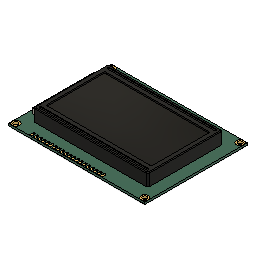
model (Autodesk Fusion 360 design; units mm, degrees)
Autodesk Fusion 360 part; units mm, degrees
note: some values were not read from the file. Set by a fixed rule: which face or edge a step refers to.
sketch "Sketch1" plane through (0, 0, 0) normal (0, 1, 0) x (1, 0, 0)
  line L0 (46.5, 35) -> (-46.5, 35)
  line L1 (-46.5, 35) -> (-46.5, -35)
  line L2 (-46.5, -35) -> (46.5, -35)
  line L3 (46.5, -35) -> (46.5, 35)
  circle A0 centre (-44, 32.5) radius 1.5
  circle A1 centre (44, 32.5) radius 1.5
  circle A2 centre (-44, -32.5) radius 1.5
  circle A3 centre (44, -32.5) radius 1.5
  line L4 (39, 25.5) -> (-39, 25.5)
  line L5 (-39, 25.5) -> (-39, -25.5)
  line L6 (-39, -25.5) -> (39, -25.5)
  line L7 (39, -25.5) -> (39, 25.5)
  line L8 (44, 21.25) -> (39, 21.25)
  line L9 (44, -21.25) -> (39, -21.25)
  line L10 (44, 21.25) -> (44, -21.25)
  dimension "d1" = 93
  dimension "d2" = 70
  dimension "d3" = 88
  dimension "d4" = 65
  dimension "d5" = 3
  dimension "d6" = 3
  dimension "d7" = 3
  dimension "d8" = 3
  dimension "d9" = 78
  dimension "d10" = 51
  constraint horizontal L0
  constraint perpendicular L0 L1
  constraint parallel L0 L2
  constraint parallel L1 L3
  constraint horizontal L4
  constraint perpendicular L4 L5
  constraint parallel L4 L6
  constraint parallel L5 L7
  constraint coincident L7 L8.end
  constraint perpendicular L7 L8
  constraint perpendicular L8 L10
  measures "d1" distance of L1.end L2.end
  measures "d2" distance of L0.end L1.end
  measures "d3" distance of A2.centre A3.centre
  measures "d4" distance of A0.centre A2.centre
  measures "d5" diameter of A0
  measures "d6" diameter of A1
  measures "d7" diameter of A2
  measures "d8" diameter of A3
  measures "d9" distance of L5.end L6.end
  measures "d10" distance of L4.end L5.end
extrude "Extrude1" add sketch "Sketch1" against normal blind 1.5 contours L0 L1 L2 L3 | L4 L5 L6 L7 | L7 L8 L9 L10 makes body 1
extrude "Extrude2" add sketch "Sketch1" along normal blind 8.5 contours L4 L5 L6 L7 bodies 1
extrude "Extrude3" add sketch "Sketch1" along normal blind 3.5 separate body contours L7 L8 L9 L10 makes body 2
extrude "Extrude4" cut 1 faces at (39, 1.1667, 7.0833) along direction (-1, 0, 0) blind 74 on bodies 2 bodies 1
split "Split1" by plane through (0, 0, 0) normal (0, 1, 0) bodies 1 makes body 3 at (-13, 8.5, -8.5)
extrude "Extrude5" cut 1 faces at (14.3333, 3.5, 7.0833) along direction (0, 1, 0) blind 1 on bodies 3 bodies 3
extrude "Extrude6" cut 1 faces at (14.3333, 1.5, -21.25) along direction (0, 0, -1) blind 1 on bodies 3 bodies 3
extrude "Extrude7" cut 1 faces at (14.3333, 1.5, 21.25) along direction (0, 0, 1) blind 1 on bodies 3 bodies 3
extrude "Extrude8" cut 1 faces at (-35, 1.5, -7.4167) along direction (-1, 0, 0) blind 0.75 on bodies 3 bodies 3
extrude "Extrude9" add 1 faces at (39, 1.1667, 7.0833) along direction (-1, 0, 0) blind 73.75 on bodies 2 bodies 2
sketch "Sketch2" plane through (0, 8.5, 0) normal (0, 1, 0) x (-1, 0, 0)
  line L0 (-39, 25.5) -> (-39, -25.5)
  line L1 (-39, -25.5) -> (39, -25.5)
  line L2 (39, -25.5) -> (39, 25.5)
  line L3 (39, 25.5) -> (-39, 25.5)
  line L4 (-35, -20) -> (35, -20)
  line L5 (36, -19) -> (36, 19)
  line L6 (35, 20) -> (-35, 20)
  line L7 (-36, 19) -> (-36, -19)
  line L8 (-36, -20) -> (36, 20) construction
  line L9 (36, -20) -> (-36, 20) construction
  arc A0 (35, -20) -> (36, -19) centre (35, -19) ccw
  arc A1 (36, 19) -> (35, 20) centre (35, 19) ccw
  arc A2 (-35, 20) -> (-36, 19) centre (-35, 19) ccw
  arc A3 (-36, -19) -> (-35, -20) centre (-35, -19) ccw
  dimension "d31" = 72
  dimension "d32" = 40
  dimension "d33" = 1
  constraint horizontal L4
  constraint perpendicular L4 L5
  constraint parallel L4 L6
  constraint parallel L5 L7
  constraint coincident L8 origin
  constraint coincident L9 origin
  constraint coincident L9.start L5
  constraint coincident L9.start L4
  constraint tangent L5 A0
  constraint tangent L4 A0
  constraint coincident L8.end L5
  constraint coincident L8.end L6
  constraint tangent L5 A1
  constraint tangent L6 A1
  constraint equal A0 A1
  constraint coincident L9.end L6
  constraint coincident L9.end L7
  constraint tangent L6 A2
  constraint tangent L7 A2
  constraint equal A0 A2
  constraint coincident L8.start L7
  constraint coincident L8.start L4
  constraint tangent L7 A3
  constraint tangent L4 A3
  constraint equal A0 A3
  measures "d31" distance of L8.end L9.end
  measures "d32" distance of L9.start L8.end
  measures "d33" radius of A0
extrude "Extrude10" cut sketch "Sketch2" against normal blind 1 contours L4 L5 L6 L7 A0 A1 A2 A3 bodies 3
chamfer "Chamfer1" distance 1 angle 45 4 edges at (-39, 4.25, 25.5) (39, 4.25, 25.5) (-39, 4.25, -25.5) (39, 4.25, -25.5) on bodies 3
fillet "Fillet1" radius 0.5 8 edges at (39, 8.5, 0) (0, 8.5, 25.5) (38.5, 8.5, 25) (38.5, 8.5, -25) (0, 8.5, -25.5) (-38.5, 8.5, 25) (-39, 8.5, 0) (-38.5, 8.5, -25) on bodies 3
sketch "Sketch3" plane through (0, 8.5, 0) normal (0, 1, 0) x (-1, 0, 0)
  line L0 (35, -20) -> (-35, -20)
  arc A0 (-36, -19) -> (-35, -20) centre (-35, -19) ccw
  line L1 (-36, -19) -> (-36, 19)
  arc A1 (-35, 20) -> (-36, 19) centre (-35, 19) ccw
  line L2 (-35, 20) -> (35, 20)
  arc A2 (36, 19) -> (35, 20) centre (35, 19) ccw
  line L3 (36, 19) -> (36, -19)
  arc A3 (35, -20) -> (36, -19) centre (35, -19) ccw
  line L4 (38.5, -24.2929) -> (38.5, 24.2929)
  line L5 (38.5, 24.2929) -> (37.7929, 25)
  line L6 (37.7929, 25) -> (-37.7929, 25)
  line L7 (-37.7929, 25) -> (-38.5, 24.2929)
  line L8 (-38.5, 24.2929) -> (-38.5, -24.2929)
  line L9 (-38.5, -24.2929) -> (-37.7929, -25)
  line L10 (-37.7929, -25) -> (37.7929, -25)
  line L11 (37.7929, -25) -> (38.5, -24.2929)
  line L12 (-36.5, -23.95) -> (36.5, -23.95)
  arc A4 (36.5, -23.95) -> (36.5, -22.45) centre (36.5, -23.2) ccw
  line L13 (36.5, -22.45) -> (-36.5, -22.45)
  arc A5 (-36.5, -22.45) -> (-36.5, -23.95) centre (-36.5, -23.2) ccw
  line L14 (-36.5, -23.2) -> (36.5, -23.2) construction
  line L15 (36.5, 23.95) -> (-36.5, 23.95)
  arc A6 (-36.5, 23.95) -> (-36.5, 22.45) centre (-36.5, 23.2) ccw
  line L16 (-36.5, 22.45) -> (36.5, 22.45)
  arc A7 (36.5, 22.45) -> (36.5, 23.95) centre (36.5, 23.2) ccw
  point P0 (0, -23.2)
  dimension "d39" = 1.5
  dimension "d40" = 1.5
  constraint tangent L12 A4
  constraint tangent A4 L13
  constraint parallel L12 L13
  constraint tangent L13 A5
  constraint tangent L12 A5
  constraint perpendicular L4 L14
  constraint midpoint L14 P0
  constraint tangent L15 A6
  constraint tangent A6 L16
  constraint parallel L15 L16
  constraint tangent L16 A7
  constraint tangent L15 A7
  measures "d39" diameter of A4
  measures "d40" diameter of A6
extrude "Extrude11" cut sketch "Sketch3" against normal blind 0.5 contours L12 A4 L13 A5 | L15 A6 L16 A7 bodies 3
cylinder "CylinderPrimitive1" add diameter 5 height 0.25 placed x (1, 0, 0) y (0, 0, -1) z (0, 1, 0) at (44, 0, 32.5) separate body makes body 4
extrude "Extrude12" add 1 faces at (43.4804, 0.25, 32.0179) along direction (0, -1, 0) blind 2 separate body on bodies 4 makes body 5
copy_body "CopyPasteBodies1" bodies 5 makes body 6
move_body "Move1" bodies 6 to x (1, 0, 0) y (0, 1, 0) z (0, 0, 1) at (-88, 0, 0)
copy_body "CopyPasteBodies2" bodies 6 5 makes body 7 makes body 8
move_body "Move2" bodies 7 8 to x (1, 0, 0) y (0, 1, 0) z (0, 0, 1) at (0, 0, -65)
combine "Combine1" operation add target body 8 tool bodies 7 6 5 4 1
cylinder "CylinderPrimitive2" cut diameter 3 height -2 placed x (1, 0, 0) y (0, 0, -1) z (0, 1, 0) at (-44, 0.25, 32.5) bodies 8
cylinder "CylinderPrimitive3" cut diameter 3 height -2 placed x (1, 0, 0) y (0, 0, -1) z (0, 1, 0) at (44, 0.25, 32.5) bodies 8
cylinder "CylinderPrimitive4" cut diameter 3 height -2 placed x (1, 0, 0) y (0, 0, -1) z (0, 1, 0) at (44, 0.25, -32.5) bodies 8
cylinder "CylinderPrimitive5" cut diameter 3 height -2 placed x (1, 0, 0) y (0, 0, -1) z (0, 1, 0) at (-44, 0.25, -32.5) bodies 8
extrude "Extrude13" cut 4 faces at (-41.8482, 0.25, -32.3013) (46.1518, 0.25, -32.3013) (46.1518, 0.25, 32.6987) (-41.8482, 0.25, 32.6987) along direction (0, -1, 0) blind 0.15 on bodies 8 bodies 8
extrude "Extrude14" cut 4 faces at (46.1518, -1.75, -32.3013) (46.1518, -1.75, 32.6987) (-41.8482, -1.75, 32.6987) (-41.8482, -1.75, -32.3013) along direction (0, 1, 0) blind 0.15 on bodies 8 bodies 8
move_body "Move3" bodies 2 8 3 to x (-1, 0, 0) y (0, 1, 0) z (0, 0, -1) at (0, 0, 0)
sketch "Sketch9" plane through (0, 0, 0) normal (0, 1, 0) x (-1, 0, 0)
  arc A0 (46.5, -32.5) -> (44, -35) centre (44, -32.5) ccw
  line L0 (46.5, -32.5) -> (46.5, 32.5)
  arc A1 (44, 35) -> (46.5, 32.5) centre (44, 32.5) ccw
  line L1 (44, 35) -> (-44, 35)
  arc A2 (-46.5, 32.5) -> (-44, 35) centre (-44, 32.5) ccw
  line L2 (-46.5, 32.5) -> (-46.5, -32.5)
  arc A3 (-44, -35) -> (-46.5, -32.5) centre (-44, -32.5) ccw
  line L3 (-44, -35) -> (44, -35)
  line L4 (46.5, 35) -> (33, 35)
  circle A4 centre (31.73, 32.7) radius 0.5
  line L5 (30.98, 32.7) -> (30.98, 34.7)
  line L6 (30.98, 34.7) -> (32.48, 34.7)
  line L7 (32.48, 32.7) -> (32.48, 34.7)
  arc A5 (30.98, 32.7) -> (32.48, 32.7) centre (31.73, 32.7) ccw
  dimension "d59" = 13.5
  constraint parallel L1 L4
  constraint concentric A4 A5
  constraint perpendicular L1 L5
  constraint perpendicular L5 L6
  measures "d59" distance of L4.start L4.end
extrude "Extrude15" add sketch "Sketch9" along normal blind 0.1 contours L5 L6 L7 A5 bodies 8
extrude "Extrude16" add 1 faces at (-31.7175, 0.1, 34.1995) along direction (0, -1, 0) blind 1.7 separate body on bodies 8 makes body 9
copy_body "CopyPasteBodies3" bodies 9 makes body 10
move_body "Move4" bodies 10 to x (1, 0, 0) y (0, 1, 0) z (0, 0, 1) at (2.54, 0, 0)
copy_body "CopyPasteBodies4" bodies 10 9 makes body 11 makes body 12
move_body "Move5" bodies 11 12 to x (1, 0, 0) y (0, 1, 0) z (0, 0, 1) at (5.08, 0, 0)
copy_body "CopyPasteBodies5" bodies 9 10 11 12 makes body 13 makes body 14 makes body 15 makes body 16
move_body "Move6" bodies 13 14 15 16 to x (1, 0, 0) y (0, 1, 0) z (0, 0, 1) at (10.16, 0, 0)
copy_body "CopyPasteBodies6" bodies 10 11 12 13 14 15 16 9 makes body 17 makes body 18 makes body 19 makes body 20 makes body 21 makes body 22 makes body 23 makes body 24
move_body "Move7" bodies 17 18 19 20 21 22 23 24 to x (1, 0, 0) y (0, 1, 0) z (0, 0, 1) at (20.23, 0, 0)
copy_body "CopyPasteBodies7" bodies 21 22 23 20 makes body 25 makes body 26 makes body 27 makes body 28
move_body "Move8" bodies 25 26 27 28 to x (1, 0, 0) y (0, 1, 0) z (0, 0, 1) at (10.16, 0, 0)
combine "Combine2" operation add target body 28 tool bodies 9 27 19 16 13 21 22 20 15 24 11 23 18 26 17 8 12 14 25 10
delete_face "DeleteFace1" 1 faces at (-31.8655, 0, 32.7248) on bodies 28
delete_face "DeleteFace2" 5 faces at (-29.0861, 0, 32.5697) (-26.5461, 0, 32.5697) (-24.0061, 0, 32.5697) (-21.7293, 0, 32.7006) (-19.1893, 0, 32.7006) on bodies 28
delete_face "DeleteFace3" 14 faces at (-16.6474, 0, 32.6757) (-14.0539, 0, 32.88) (-11.6039, 0, 32.88) (-9.0639, 0, 32.88) (-6.5184, 0, 32.9043) (-4.0022, 0, 32.863) (-1.4439, 0, 32.88) (1.0961, 0, 32.88) (3.6361, 0, 32.88) (6.1816, 0, 32.9043) (11.2561, 0, 32.88) (8.7161, 0, 32.88) (13.7961, 0, 32.88) (16.3361, 0, 32.88) on bodies 28
sketch "Sketch10" plane through (0, 0, 0) normal (1, 0, 0) x (0, 0, -1)
  line L0 (0, -1.5) -> (0, -2.5)
  line L1 (0, -1.5) -> (7.5, -1.5)
  arc A0 (0, -2.5) -> (7.5, -1.5) centre (0, 26.125) ccw
  dimension "d71" = 7.5
  constraint vertical L0
  constraint perpendicular L0 L1
  measures "d71" distance of L0.start L1.end
revolve "Revolve1" add sketch "Sketch10" angle 360 about axis through (0, 1.75, 0) along (0, 1, 0) separate body makes body 29
sketch "Sketch11" plane through (0, -1.5, 0) normal (0, -1, 0) x (1, 0, 0)
  arc A0 (10.61, 32.7) -> (12.11, 32.7) centre (11.36, 32.7) ccw
  line L0 (10.61, 32.7) -> (10.61, 34.7)
  line L1 (10.61, 34.7) -> (12.11, 34.7)
  line L2 (12.11, 34.7) -> (12.11, 32.7)
  arc A1 (-27.4, 32.7) -> (-25.9, 32.7) centre (-26.65, 32.7) ccw
  line L3 (-27.4, 32.7) -> (-27.4, 34.7)
  line L4 (-27.4, 34.7) -> (-25.9, 34.7)
  line L5 (-25.9, 34.7) -> (-25.9, 32.7)
  arc A2 (15.69, 32.7) -> (17.19, 32.7) centre (16.44, 32.7) ccw
  line L6 (15.69, 32.7) -> (15.69, 34.7)
  line L7 (15.69, 34.7) -> (17.19, 34.7)
  line L8 (17.19, 34.7) -> (17.19, 32.7)
  arc A3 (2.99, 32.7) -> (4.49, 32.7) centre (3.74, 32.7) ccw
  line L9 (2.99, 32.7) -> (2.99, 34.7)
  line L10 (2.99, 34.7) -> (4.49, 34.7)
  line L11 (4.49, 34.7) -> (4.49, 32.7)
  arc A4 (-12.25, 32.7) -> (-10.75, 32.7) centre (-11.5, 32.7) ccw
  line L12 (-12.25, 32.7) -> (-12.25, 34.7)
  line L13 (-12.25, 34.7) -> (-10.75, 34.7)
  line L14 (-10.75, 34.7) -> (-10.75, 32.7)
  arc A5 (-2.09, 32.7) -> (-0.59, 32.7) centre (-1.34, 32.7) ccw
  line L15 (-2.09, 32.7) -> (-2.09, 34.7)
  line L16 (-2.09, 34.7) -> (-0.59, 34.7)
  line L17 (-0.59, 34.7) -> (-0.59, 32.7)
  arc A6 (0.45, 32.7) -> (1.95, 32.7) centre (1.2, 32.7) ccw
  line L18 (0.45, 32.7) -> (0.45, 34.7)
  line L19 (0.45, 34.7) -> (1.95, 34.7)
  line L20 (1.95, 34.7) -> (1.95, 32.7)
  arc A7 (-17.24, 32.7) -> (-15.74, 32.7) centre (-16.49, 32.7) ccw
  line L21 (-17.24, 32.7) -> (-17.24, 34.7)
  line L22 (-17.24, 34.7) -> (-15.74, 34.7)
  line L23 (-15.74, 34.7) -> (-15.74, 32.7)
  arc A8 (13.15, 32.7) -> (14.65, 32.7) centre (13.9, 32.7) ccw
  line L24 (13.15, 32.7) -> (13.15, 34.7)
  line L25 (13.15, 34.7) -> (14.65, 34.7)
  line L26 (14.65, 34.7) -> (14.65, 32.7)
  arc A9 (8.07, 32.7) -> (9.57, 32.7) centre (8.82, 32.7) ccw
  line L27 (8.07, 32.7) -> (8.07, 34.7)
  line L28 (8.07, 34.7) -> (9.57, 34.7)
  line L29 (9.57, 34.7) -> (9.57, 32.7)
  arc A10 (-32.48, 32.7) -> (-30.98, 32.7) centre (-31.73, 32.7) ccw
  line L30 (-32.48, 32.7) -> (-32.48, 34.7)
  line L31 (-32.48, 34.7) -> (-30.98, 34.7)
  line L32 (-30.98, 34.7) -> (-30.98, 32.7)
  arc A11 (-7.17, 32.7) -> (-5.67, 32.7) centre (-6.42, 32.7) ccw
  line L33 (-7.17, 32.7) -> (-7.17, 34.7)
  line L34 (-7.17, 34.7) -> (-5.67, 34.7)
  line L35 (-5.67, 34.7) -> (-5.67, 32.7)
  arc A12 (-22.32, 32.7) -> (-20.82, 32.7) centre (-21.57, 32.7) ccw
  line L36 (-22.32, 32.7) -> (-22.32, 34.7)
  line L37 (-22.32, 34.7) -> (-20.82, 34.7)
  line L38 (-20.82, 34.7) -> (-20.82, 32.7)
  arc A13 (5.53, 32.7) -> (7.03, 32.7) centre (6.28, 32.7) ccw
  line L39 (5.53, 32.7) -> (5.53, 34.7)
  line L40 (5.53, 34.7) -> (7.03, 34.7)
  line L41 (7.03, 34.7) -> (7.03, 32.7)
  arc A14 (-14.7, 32.7) -> (-13.2, 32.7) centre (-13.95, 32.7) ccw
  line L42 (-14.7, 32.7) -> (-14.7, 34.7)
  line L43 (-14.7, 34.7) -> (-13.2, 34.7)
  line L44 (-13.2, 34.7) -> (-13.2, 32.7)
  arc A15 (-24.86, 32.7) -> (-23.36, 32.7) centre (-24.11, 32.7) ccw
  line L45 (-24.86, 32.7) -> (-24.86, 34.7)
  line L46 (-24.86, 34.7) -> (-23.36, 34.7)
  line L47 (-23.36, 34.7) -> (-23.36, 32.7)
  arc A16 (-4.63, 32.7) -> (-3.13, 32.7) centre (-3.88, 32.7) ccw
  line L48 (-4.63, 32.7) -> (-4.63, 34.7)
  line L49 (-4.63, 34.7) -> (-3.13, 34.7)
  line L50 (-3.13, 34.7) -> (-3.13, 32.7)
  arc A17 (-9.71, 32.7) -> (-8.21, 32.7) centre (-8.96, 32.7) ccw
  line L51 (-9.71, 32.7) -> (-9.71, 34.7)
  line L52 (-9.71, 34.7) -> (-8.21, 34.7)
  line L53 (-8.21, 34.7) -> (-8.21, 32.7)
  arc A18 (-44, -35) -> (-46.5, -32.5) centre (-44, -32.5) ccw
  line L54 (-44, -35) -> (44, -35)
  arc A19 (46.5, -32.5) -> (44, -35) centre (44, -32.5) ccw
  line L55 (46.5, -32.5) -> (46.5, 32.5)
  arc A20 (44, 35) -> (46.5, 32.5) centre (44, 32.5) ccw
  line L56 (44, 35) -> (-44, 35)
  arc A21 (-46.5, 32.5) -> (-44, 35) centre (-44, 32.5) ccw
  line L57 (-46.5, 32.5) -> (-46.5, -32.5)
  arc A22 (-19.78, 32.7) -> (-18.28, 32.7) centre (-19.03, 32.7) ccw
  line L58 (-19.78, 32.7) -> (-19.78, 34.7)
  line L59 (-19.78, 34.7) -> (-18.28, 34.7)
  line L60 (-18.28, 34.7) -> (-18.28, 32.7)
  arc A23 (-29.94, 32.7) -> (-28.44, 32.7) centre (-29.19, 32.7) ccw
  line L61 (-29.94, 32.7) -> (-29.94, 34.7)
  line L62 (-29.94, 34.7) -> (-28.44, 34.7)
  line L63 (-28.44, 34.7) -> (-28.44, 32.7)
  circle A24 centre (21.5, -10) radius 7.5
  circle A25 centre (6.5, 9) radius 7.5
  circle A26 centre (-18.5, -9) radius 7.5
  dimension "d75" = 15
  dimension "d78" = 15
  dimension "d81" = 15
  measures "d75" diameter of A24
  measures "d78" diameter of A25
  measures "d81" diameter of A26
move_body "Move9" bodies 29 to x (1, 0, 0) y (0, 1, 0) z (0, 0, 1) at (-18.5, 0, -9)
copy_body "CopyPasteBodies8" bodies 29 makes body 30
move_body "Move10" bodies 30 to x (1, 0, 0) y (0, 1, 0) z (0, 0, 1) at (25, 0, 18)
copy_body "CopyPasteBodies9" bodies 29 makes body 31
move_body "Move11" bodies 31 to x (1, 0, 0) y (0, 1, 0) z (0, 0, 1) at (40, 0, -1)
combine "Combine3" operation add target body 28 tool bodies 29 30 31
named bodies: "backlight", "display", "pcb"
